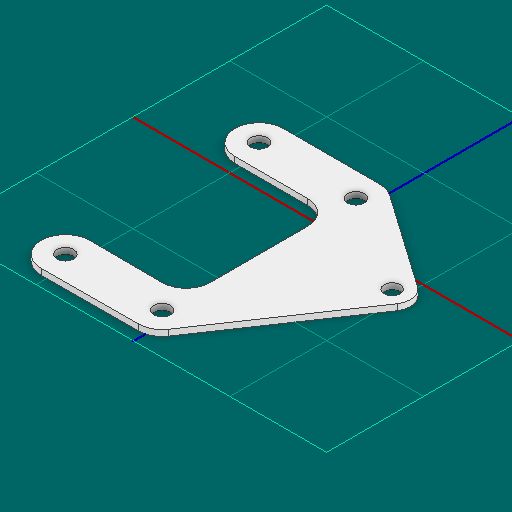
# Autodesk Inventor part: gusset
Saved by Autodesk Inventor 2025 (Build 290162000, 162)
## iProperties
Created: 2024-09-29
Part Number: gusset
Material: Acetal Resin, White
Document SubType Name: Modeling
Designer: averey
Density: 1.425 g/cm^3
Appearance: Smooth - White
Author: averey
Autodesk Inventor part; units mm, degrees
ref_plane "YZ Plane" through (0, 0, 0) normal (1, 0, 0) x (0, 1, 0)
ref_plane "XZ Plane" through (0, 0, 0) normal (0, 1, 0) x (-1, 0, 0)
ref_plane "XY Plane" through (0, 0, 0) normal (0, 0, 1) x (1, 0, 0)
sketch "Sketch1" plane through (0, 0, 0) normal (0, 1, 0) x (-1, 0, 0)
  circle A0 centre (1.4772, 41.6579) radius 2.1844
  circle A1 centre (26.8772, 41.6579) radius 2.1844
  circle A2 centre (26.8772, -9.1421) radius 2.1844
  circle A3 centre (1.4772, -9.1421) radius 2.1844
  arc A4 (1.4487, 47.8916) -> (-3.6864, 45.1505) centre (1.4772, 41.6579) ccw
  arc A5 (26.8481, 35.3079) -> (26.8191, 48.0076) centre (26.8772, 41.6579) ccw
  arc A6 (26.8487, -15.4921) -> (26.8487, -2.7922) centre (26.8772, -9.1421) ccw
  circle A7 centre (-23.9228, 6.7329) radius 2.0955
  arc A8 (-27.8677, 9.4012) -> (-26.6575, 2.8337) centre (-23.9228, 6.7329) ccw
  line L0 (-3.6864, 45.1505) -> (-27.8677, 9.4012)
  line L1 (-26.6575, 2.8337) -> (-2.169, -14.341)
  line L2 (26.8772, 48.0079) -> (1.4487, 47.8916)
  line L3 (26.8481, 35.3079) -> (7.8277, 35.3949)
  line L4 (1.4487, 29.045) -> (1.4487, 3.5578)
  line L5 (26.9057, -2.7922) -> (7.7987, -2.7922)
  line L6 (26.9057, -15.4921) -> (1.4487, -15.4921)
  arc A9 (1.5057, -2.7922) -> (1.4487, -2.7922) centre (1.4772, -9.1421) ccw
  arc A10 (-2.169, -14.341) -> (1.5057, -15.4921) centre (1.4772, -9.1421) ccw
  arc A11 (7.8277, 35.3949) -> (1.4487, 29.045) centre (7.7987, 29.045) ccw
  arc A12 (1.4487, 3.5578) -> (7.7987, -2.7922) centre (7.7987, 3.5578) ccw
  point P0 (0, 0)
  dimension "d0" = 4.191
  dimension "d1" = 9.525
  dimension "d2" = 25.4
  dimension "d3" = 6.35
  constraints: 20 point on circle, 14 end point, 13 centre point, 11 tangent, 8 point on line, 5 coincident, 1 equal radius, 1 perpendicular, 1 vertical, 2 other
  measures "d0" diameter of A7
  measures "d1" diameter of A8
  measures "d2" horizontal distance of A7.centre A3.centre
  measures "d3" radius of A11
extrude "Extrusion1" add sketch "Sketch1" along normal blind 1.5875
body "Solid1"
